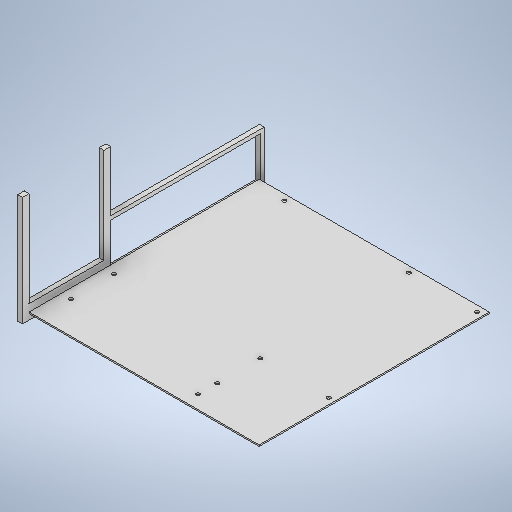
# Autodesk Inventor part: matx-arc-case-r2
Saved by Autodesk Inventor 2025 (Build 290162000, 162)
## iProperties
Created: 2024-07-20
Part Number: matx-arc-case-r2
Material: Generic
Document SubType Name: Modeling
Designer: admin
Density: 1 g/cm^3
Appearance: Default
Author: admin
Autodesk Inventor part; units mm, degrees
ref_plane "YZ Plane" through (0, 0, 0) normal (1, 0, 0) x (0, 1, 0)
ref_plane "XZ Plane" through (0, 0, 0) normal (0, 1, 0) x (-1, 0, 0)
ref_plane "XY Plane" through (0, 0, 0) normal (0, 0, 1) x (1, 0, 0)
sketch "Sketch1" plane through (0, 0, 0) normal (0, 1, 0) x (-1, 0, 0)
  line L0 (0, 0) -> (0, -244)
  line L1 (0, -244) -> (244, -244)
  line L2 (244, -244) -> (244, 0)
  line L3 (244, 0) -> (0, 0)
  line L4 (0, 0) -> (0, -22.86)
  line L5 (0, -22.86) -> (0, -177.8)
  line L6 (0, 0) -> (0, -227.33)
  line L7 (0, 0) -> (0, -154.94)
  line L8 (0, 0) -> (6.25, 0)
  line L9 (0, 0) -> (158.75, 0)
  circle A0 centre (0, -22.86) radius 3
  circle A1 centre (0, -154.94) radius 3
  circle A2 centre (0, -227.33) radius 3
  line L10 (0, -227.33) -> (203.2, -227.33)
  circle A3 centre (200.2, -151.94) radius 3
  line L11 (203.2, -227.33) -> (157.48, -227.33)
  circle A4 centre (157.48, -227.33) radius 3
  circle A5 centre (157.48, -151.94) radius 3
  line L12 (200.2, -151.94) -> (234.49, -151.94)
  circle A6 centre (234.49, -151.94) radius 3
  circle A7 centre (203.2, 0) radius 3
  circle A8 centre (157.48, 0) radius 3
  dimension "d35" = 244
  dimension "d36" = 244
  dimension "d37" = 244
  dimension "d38" = 244
  dimension "d62" = 22.86
  dimension "d64" = 227.33
  dimension "d65" = 154.94
  dimension "d67" = 158.75
  dimension "d68" = 6
  dimension "d69" = 6
  dimension "d70" = 6
  dimension "d71" = 203.2
  dimension "d73" = 6
  dimension "d75" = 45.72
  dimension "d76" = 34.29
  dimension "d77" = 6
  dimension "d78" = 6
  constraints: 26 end point, 9 centre point, 8 point on line, 6 coincident, 3 perpendicular, 1 horizontal, 1 vertical
  measures "d35" distance of L0.start L0.end
  measures "d36" distance of L0.end L1.end
  measures "d37" distance of L1.end L2.end
  measures "d38" distance of L2.end L0.start
  measures "d62" distance of L0.start L4.end
  measures "d64" distance of L0.start L6.end
  measures "d65" distance of L0.start L7.end
  measures "d67" distance of L0.start L9.end
  measures "d68" diameter of A0
  measures "d69" diameter of A1
  measures "d70" diameter of A2
  measures "d71" distance of L10.start L10.end
  measures "d73" diameter of A3
  measures "d75" distance of L11.start L11.end
  measures "d76" distance of L12.start L12.end
  measures "d77" diameter of A7
  measures "d78" diameter of A8
sketch "Sketch2" plane through (0, 0, 0) normal (0, 1, 0) x (-1, 0, 0)
  line L0 (0, 0) -> (0, -243.84)
  line L1 (0, -243.84) -> (243.84, -243.84)
  line L2 (243.84, -243.84) -> (243.84, 0)
  line L3 (243.84, 0) -> (0, 0)
  line L4 (243.84, 0) -> (233.68, 0)
  line L5 (233.68, 0) -> (6.35, 0)
  line L6 (233.68, 0) -> (78.74, 0)
  line L7 (233.68, -243.84) -> (210.82, -243.84)
  line L8 (233.68, 0) -> (233.68, -243.84)
  line L9 (243.84, -243.84) -> (243.84, -85.09)
  line L10 (6.35, 0) -> (6.35, -243.84)
  line L11 (78.74, 0) -> (78.74, -243.84)
  line L12 (243.84, -85.09) -> (243.84, -31.85)
  line L13 (78.74, -31.85) -> (78.74, -77.57)
  line L14 (78.74, 0) -> (78.74, -34.29)
  line L15 (78.74, -34.29) -> (78.74, -13.97)
  line L16 (78.74, -34.29) -> (78.74, -80.01)
  circle A0 centre (78.74, -80.01) radius 2
  circle A1 centre (78.74, -34.29) radius 2
  circle A2 centre (78.74, -13.97) radius 2
  circle A3 centre (6.35, -80.01) radius 2
  line L17 (78.74, -34.29) -> (78.74, -237.49)
  circle A4 centre (78.74, -237.49) radius 2
  circle A5 centre (6.35, -237.49) radius 2
  circle A6 centre (210.82, -237.49) radius 2
  circle A7 centre (233.68, -34.29) radius 2
  circle A8 centre (233.68, -80.01) radius 2
  dimension "d79" = 243.84
  dimension "d80" = 243.84
  dimension "d81" = 10.16
  dimension "d82" = 227.33
  dimension "d83" = 154.94
  dimension "d84" = 22.86
  dimension "d85" = 158.75
  dimension "d92" = 34.29
  dimension "d93" = 20.32
  dimension "d94" = 45.72
  dimension "d95" = 203.2
  constraints: 36 end point, 17 point on line, 9 centre point, 4 coincident, 4 perpendicular, 2 vertical, 1 parallel
  measures "d79" distance of L0.start L0.end
  measures "d80" distance of L0.end L1.end
  measures "d81" distance of L2.end L4.end
  measures "d82" distance of L4.end L5.end
  measures "d83" distance of L4.end L6.end
  measures "d84" distance of L7.start L7.end
  measures "d85" distance of L1.end L9.end
  measures "d92" distance of L6.end L14.end
  measures "d93" distance of L14.end L15.end
  measures "d94" distance of L14.end L16.end
  measures "d95" distance of L17.start L17.end
extrude "Extrusion1" add sketch "Sketch2" along normal blind 1.5 contours L3 L10 A3 A5 L1 L0 | L3 L11 A2 A1 A0 A4 L1 L10 A5 A3 | L3 L8 A7 A8 L1 L11 A4 A0 A1 A2 | L3 L2 L1 L8 A8 A7
sketch "Sketch4" plane through (-243.84, 0, -243.84) normal (-1, 0, 0) x (0, 0, 1)
  line L0 (0.0105, -0.4083) -> (0.0105, -1.9083)
  line L1 (243.84, 0) -> (0, 0) projected
  line L2 (0.0105, -1.9083) -> (-1.25, -1.9083)
  line L3 (-1.25, -1.9083) -> (-1.25, 42.5417)
  line L4 (-1.25, -1.9083) -> (43.2, -1.9083) construction
  line L5 (-1.25, 42.5417) -> (157.5, 42.5417)
  line L6 (157.5, 42.5417) -> (157.5, -1.9083)
  line L7 (-1.25, -1.9083) -> (-1.25, -6.0083)
  line L8 (-1.25, -6.0083) -> (157.5, -6.0083)
  line L9 (-1.25, -6.0083) -> (-5.35, -6.0083)
  line L10 (-5.35, -6.0083) -> (-5.35, 42.5417)
  line L11 (-5.35, 42.5417) -> (-5.35, 46.6417)
  line L12 (-5.35, 46.6417) -> (157.5, 46.6417)
  line L13 (157.5, 46.6417) -> (161.6, 46.6417)
  line L14 (161.6, 46.6417) -> (161.6, -1.9083)
  line L15 (161.6, -6.0083) -> (157.5, -6.0083)
  line L16 (161.6, -6.0083) -> (161.6, -1.9083)
  line L17 (0.0105, -1.9083) -> (157.5, -1.9083)
  line L18 (161.6, -6.0083) -> (243.84, -6.0083)
  line L19 (161.6, -6.0083) -> (161.6, 9.1917)
  line L20 (161.6, 9.1917) -> (243.84, 9.1917)
  line L21 (243.84, 9.1917) -> (243.84, -6.0083)
  line L22 (157.5, 42.5417) -> (164.5, 42.5417)
  line L23 (164.5, 42.5417) -> (164.5, 9.1917)
  line L24 (164.5, 42.5417) -> (164.5, 46.6417)
  line L25 (164.5, 46.6417) -> (161.6, 46.6417)
  line L26 (164.5, 9.1917) -> (164.5, 110.1917)
  line L27 (164.5, 110.1917) -> (243.84, 110.1917)
  line L28 (243.84, 110.1917) -> (243.84, 9.1917)
  line L29 (157.5, 46.6417) -> (157.5, 110.1917)
  line L30 (250.84, 110.1917) -> (250.84, -6.0083)
  line L31 (250.84, -6.0083) -> (243.84, -6.0083)
  line L32 (243.84, 110.1917) -> (250.84, 110.1917)
  line L33 (157.5, 110.1917) -> (164.5, 110.1917)
  dimension "d98" = 1.5
  dimension "d103" = 44.45
  dimension "d104" = 90
  dimension "d105" = 158.75
  dimension "d106" = 4.1
  dimension "d107" = 4.1
  dimension "d108" = 4.1
  dimension "d109" = 4.1
  dimension "d110" = 15.2
  dimension "d111" = 7
  dimension "d112" = 101
  constraints: 66 end point, 14 perpendicular, 13 point on line, 3 horizontal, 3 vertical, 2 collinear, 2 parallel
  measures "d98" distance of L0.start L0.end
  measures "d103" distance of L2.end L3.end
  measures "d104" angle of L4 L3
  measures "d105" distance of L3.end L5.end
  measures "d106" distance of L2.end L7.end
  measures "d107" distance of L7.end L9.end
  measures "d108" distance of L10.end L11.end
  measures "d109" distance of L12.end L13.end
  measures "d110" distance of L15.start L19.end
  measures "d111" distance of L5.end L22.end
  measures "d112" distance of L23.end L26.end
extrude "Extrusion2" add sketch "Sketch4" along normal blind 5 contours L21 L18 L16 L14 L1 | L1 L14 L20 L21 | L21 L28 L32 L30 L31 | L14 L16 L15 L8 L7 L2 L17 L6 L1 | L1 L6 L22 L14 | L14 L22 L23 L20 | L5 L3 L7 L9 L10 L11 L12 L13 L14 L22 | L14 L25 L24 L22 | L26 L25 L13 L29 L33
body "Solid1"
